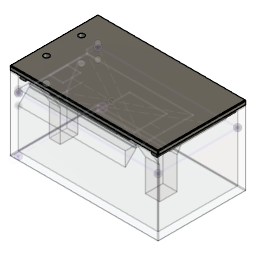
ESP32_case_v2 (Autodesk Fusion 360 design; units mm, degrees)
Autodesk Fusion 360 part; units mm, degrees
note: some values were not read from the file. Chosen so that the rebuilt part matches the saved one: a direction. Set by a fixed rule: which sketch regions a step uses.
sketch "Sketch1" plane through (0, 0, 0) normal (0, 0, 1) x (1, 0, 0) in component "Case bottom"
  line L0 (0, 0) -> (63.9, 0)
  line L1 (63.9, 0) -> (63.9, 36.4)
  line L2 (63.9, 36.4) -> (0, 36.4)
  line L3 (0, 36.4) -> (0, 0)
  line L4 (-2, -2) -> (65.9, -2)
  line L5 (65.9, -2) -> (65.9, 38.4)
  line L6 (65.9, 38.4) -> (-2, 38.4)
  line L7 (-2, 38.4) -> (-2, -2)
  dimension "d3" = 63.9
  dimension "d4" = 36.4
  dimension "d5" = 2
  constraint horizontal L0
  constraint vertical L1
  constraint horizontal L2
  constraint vertical L3
  constraint coincident L0.start L3.end
  measures "d3" distance of L0.start L0.end
  measures "d4" distance of L0.start L2.end
extrude "Extrude1" add sketch "Sketch1" along normal blind 2 contours L0 L1 L2 L3 | L4 L5 L6 L7 makes body 1 in component "Case bottom"
extrude "Extrude2" add sketch "Sketch1" along normal blind 34 bodies 1 in component "Case bottom"
sketch "Sketch2" plane through (0, 0, 0) normal (1, 0, 0) x (0, 1, 0) in component "Case bottom"
  line L0 (36.4, 2) -> (36.4, 34)
  line L1 (36.4, 34) -> (0, 34)
  line L2 (0, 34) -> (0, 2)
  line L3 (14.2, 0) -> (22.2, 0)
  line L4 (22.2, 0) -> (22.2, 14.6077)
  line L5 (22.2, 14.6077) -> (14.2, 14.6077)
  line L6 (14.2, 14.6077) -> (14.2, 0)
  line L7 (18.2, 14.6077) -> (18.2, 0) construction
  line L8 (-2, 0) -> (38.4, 0) construction
  line L9 (22.2, 14.6077) -> (28.2, 25)
  line L10 (22.2, 14.6077) -> (29.239, 14.6077) construction
  line L11 (14.2, 14.6077) -> (8.2, 25)
  line L12 (14.2, 14.6077) -> (29.239, 14.6077) construction
  line L13 (8.2, 25) -> (28.2, 25)
  line L14 (0, 2) -> (36.4, 2)
  line L15 (0, 20) -> (5, 25)
  line L16 (5, 25) -> (5, 26.5)
  line L17 (5, 26.5) -> (0, 26.5)
  line L18 (8.2, 25) -> (0, 25) construction
  line L19 (31.4, 26.5) -> (36.4, 26.5)
  line L20 (31.4, 25) -> (31.4, 26.5)
  line L21 (36.4, 20) -> (31.4, 25)
  dimension "d12" = 8
  dimension "d13" = 60
  dimension "d14" = 120
  dimension "d15" = 20
  dimension "d17" = 7.039
  dimension "d18" = 25
  dimension "d113" = 1.5
  dimension "d114" = 5
  dimension "d115" = 45
  constraint horizontal L3
  constraint vertical L4
  constraint horizontal L5
  constraint vertical L6
  constraint midpoint L5 L7.start
  constraint midpoint L3 L7.end
  constraint midpoint L7.end L8
  constraint horizontal L10
  constraint horizontal L12
  constraint horizontal L13
  constraint coincident L2 L15.start
  constraint parallel L2 L16
  constraint coincident L2 L17.end
  constraint perpendicular L2 L17
  constraint coincident L2 L18.end
  constraint perpendicular L2 L18
  constraint coincident L15.end L18
  constraint symmetric L7 L15.start L21.start
  constraint symmetric L7 L15.end L20.start
  constraint symmetric L7 L16.end L19.start
  constraint symmetric L7 L17.end L19.end
  measures "d12" distance of L4.end L5.end
  measures "d13" angle of L9 L10
  measures "d14" angle of L11 L12
  measures "d15" distance of L9.end L11.end
  measures "d17" distance of L4.end L10.end
  measures "d18" distance of L8 L11.end
  measures "d113" distance of L15.end L16.end
  measures "d114" distance of L16.end L17.end
  measures "d115" angle of L2 L15
extrude "Extrude3" add sketch "Sketch2" along normal blind 5 separate body contours L4 L5 L6 L14 | L3 L4 L6 L14 | L5 L9 L11 L13 makes body 2 in component "Case bottom"
fillet "Fillet1" radius 1 2 edges at (2.5, 28.2, 25) (2.5, 8.2, 25) on bodies 2 in component "Case bottom"
pattern_linear "R-Pattern1" count 2 spacing 43.9 along (1, 0, 0) of bodies 2 makes body 3 in component "Case bottom"
sketch "Sketch1 (2)" plane through (0, 0, 25) normal (0, 0, 1) x (-1, 0, 0) in component "board"
  line L0 (0, -9.9321) -> (-5, -9.9321)
  line L1 (-5, -9.9321) -> (-5, -26.4679)
  line L2 (-5, -26.4679) -> (0, -26.4679)
  line L3 (0, -26.4679) -> (0, -9.9321)
  line L4 (0, -36.4) -> (0, 0)
  line L5 (-63.9, -36.4) -> (0, -36.4)
  line L6 (-63.9, 0) -> (-63.9, -36.4)
  line L7 (0, 0) -> (-63.9, 0)
  line L8 (0, -36.4) -> (-63.9, 0) construction
  line L9 (-63.9, -36.4) -> (0, 0) construction
  line L10 (-48.7, -5.2) -> (-0.2, -5.2)
  line L11 (-0.2, -5.2) -> (-0.2, -31.2)
  line L12 (-0.2, -31.2) -> (-48.7, -31.2)
  line L13 (-48.7, -31.2) -> (-48.7, -5.2)
  line L14 (-48.7, -5.2) -> (-0.2, -31.2) construction
  line L15 (-0.2, -5.2) -> (-48.7, -31.2) construction
  line L16 (-25.2, -25.7) -> (-42.2, -25.7)
  line L17 (-42.2, -25.7) -> (-42.2, -10.7)
  line L18 (-42.2, -10.7) -> (-25.2, -10.7)
  line L19 (-25.2, -10.7) -> (-25.2, -25.7)
  line L20 (-42.2, -18.2) -> (-48.7, -18.2) construction
  line L21 (-0.2, -22.2) -> (-6.2, -22.2)
  line L22 (-6.2, -22.2) -> (-6.2, -14.2)
  line L23 (-6.2, -14.2) -> (-0.2, -14.2)
  line L24 (-0.2, -14.2) -> (-0.2, -22.2)
  line L25 (-6.2, -18.2) -> (-25.2, -18.2) construction
  circle A0 centre (-2.7, -26.2) radius 1.25
  circle A1 centre (-2.7, -10.2) radius 1.25
  point P0 (-24.45, -18.2)
  dimension "d32" = 48.5
  dimension "d33" = 26
  dimension "d85" = 17
  dimension "d86" = 15
  dimension "d87" = 6.5
  dimension "d89" = 6
  dimension "d90" = 8
  dimension "d124" = 2.5
  dimension "d125" = 2.5
  dimension "d126" = 5
  dimension "d127" = 5
  dimension "d128" = 2.5
  dimension "d129" = 2.5
  dimension "d141" = 5.2
  dimension "d142" = 0.2
  constraint coincident L4.start L5.end
  constraint coincident L6.start L7.end
  constraint coincident L5.start L6.end
  constraint coincident L4.end L7.start
  constraint horizontal L10
  constraint perpendicular L10 L11
  constraint parallel L10 L12
  constraint parallel L11 L13
  constraint coincident L14 P0
  constraint coincident L15 P0
  constraint horizontal L16
  constraint vertical L17
  constraint horizontal L18
  constraint vertical L19
  constraint midpoint L17 L20.start
  constraint midpoint L13 L20.end
  constraint horizontal L20
  constraint horizontal L21
  constraint vertical L22
  constraint horizontal L23
  constraint vertical L24
  constraint coincident L11 L21.start
  constraint midpoint L22 L25.start
  constraint midpoint L19 L25.end
  constraint horizontal L25
  measures "d32" distance of L11.end L12.end
  measures "d33" distance of L10.end L11.end
  measures "d85" distance of L16.start L16.end
  measures "d86" distance of L16.start L18.end
  measures "d87" distance of L13 L17
  measures "d89" distance of L21.start L21.end
  measures "d90" distance of L21.start L23.end
  measures "d124" distance of L11 A0.centre
  measures "d125" distance of L11 A1.centre
  measures "d126" distance of L12 A0.centre
  measures "d127" distance of L10 A1.centre
  measures "d128" diameter of A0
  measures "d129" diameter of A1
  measures "d141" distance of L5 L12
  measures "d142" distance of L4 L11
extrude "Extrude2'" add sketch "Sketch1 (2)" along normal blind 1.54 separate body contours L0 L1 L11 L23 A1 | L0 L1 L2 L10 L11 L12 L13 L21 L22 L23 A0 A1 | L0 A1 | L0 A1 | L1 L11 L21 L23 L24 | L1 L2 L11 L21 A0 | L1 L21 L22 L23 | L2 A0 | L2 A0 | L16 L17 L18 L19 makes body 4 in component "board"
sketch "Sketch2 (2)" plane through (0.2, 0, 0) normal (-1, 0, 0) x (0, -1, 0) in component "board"
  line L0 (-31.2, 25) -> (-5.2, 25)
  line L1 (-5.2, 25) -> (-5.2, 26.54)
  line L2 (-5.2, 26.54) -> (-31.2, 26.54)
  line L3 (-31.2, 26.54) -> (-31.2, 25)
  line L4 (-22.7, 26.54) -> (-13.7, 26.54)
  line L5 (-13.7, 26.54) -> (-13.7, 29.56)
  line L6 (-13.7, 29.56) -> (-22.7, 29.56)
  line L7 (-22.7, 29.56) -> (-22.7, 26.54)
  dimension "d36" = 9
  dimension "d37" = 3.02
  constraint horizontal L4
  constraint vertical L5
  constraint horizontal L6
  constraint vertical L7
  constraint coincident L2 L4.start
  constraint midpoint L2 L4
  measures "d36" distance of L4.start L4.end
  measures "d37" distance of L4.start L6.end
extrude "Extrude3'" add sketch "Sketch2 (2)" along normal blind 2.2 and the other way blind 6 contours L2 L4 L5 L6 L7 bodies 4 in component "board"
fillet "Fillet1'" radius 1 4 edges at (2.1, 13.7, 29.56) (-0.9, 13.7, 26.54) (2.1, 22.7, 29.56) (-0.9, 22.7, 26.54) on bodies 4 in component "board"
sketch "Sketch3" plane through (-2, 0, 0) normal (-1, 0, 0) x (0, -1, 0) in component "Case bottom"
  line L0 (-38.4, 0) -> (2, 0)
  line L1 (2, 0) -> (2, 34)
  line L2 (2, 34) -> (-38.4, 34)
  line L3 (-38.4, 34) -> (-38.4, 0)
  arc A0 (-22.7, 27.54) -> (-21.7, 26.54) centre (-21.7, 27.54) ccw
  line L4 (-21.7, 26.54) -> (-14.7, 26.54)
  arc A1 (-14.7, 26.54) -> (-13.7, 27.54) centre (-14.7, 27.54) ccw
  line L5 (-13.7, 27.54) -> (-13.7, 28.56)
  arc A2 (-13.7, 28.56) -> (-14.7, 29.56) centre (-14.7, 28.56) ccw
  line L6 (-14.7, 29.56) -> (-21.7, 29.56)
  arc A3 (-21.7, 29.56) -> (-22.7, 28.56) centre (-21.7, 28.56) ccw
  line L7 (-22.7, 28.56) -> (-22.7, 27.54)
  line L8 (-23.7, 28.56) -> (-23.7, 27.54)
  arc A4 (-23.7, 27.54) -> (-21.7, 25.54) centre (-21.7, 27.54) ccw
  line L9 (-21.7, 25.54) -> (-14.7, 25.54)
  arc A5 (-14.7, 25.54) -> (-12.7, 27.54) centre (-14.7, 27.54) ccw
  line L10 (-12.7, 27.54) -> (-12.7, 28.56)
  arc A6 (-12.7, 28.56) -> (-14.7, 30.56) centre (-14.7, 28.56) ccw
  line L11 (-14.7, 30.56) -> (-21.7, 30.56)
  arc A7 (-21.7, 30.56) -> (-23.7, 28.56) centre (-21.7, 28.56) ccw
  dimension "d44" = 1
extrude "Extrude4" cut sketch "Sketch3" against normal blind 2 contours A0 L4 A1 L5 A2 L6 A3 L7 | L8 A4 L9 A5 L10 A6 L11 A7 bodies 1 in component "Case bottom"
sketch "Sketch1 (3)" plane through (0, 0, 34) normal (0, 0, 1) x (-1, 0, 0) in component "Lid"
  line L0 (0, 0) -> (0, -36.4)
  line L1 (0, -36.4) -> (-63.9, -36.4)
  line L2 (-63.9, -36.4) -> (-63.9, 0)
  line L3 (-63.9, 0) -> (0, 0)
  line L4 (2, -38.4) -> (2, 2)
  line L5 (2, 2) -> (-65.9, 2)
  line L6 (-65.9, 2) -> (-65.9, -38.4)
  line L7 (-65.9, -38.4) -> (2, -38.4)
  line L8 (-13.95, -36.2) -> (-49.95, -36.2)
  line L9 (-49.95, -36.2) -> (-49.95, -33.2)
  line L10 (-49.95, -33.2) -> (-13.95, -33.2)
  line L11 (-13.95, -33.2) -> (-13.95, -36.2)
  line L12 (-63.9, -36.4) -> (0, -36.4)
  line L13 (-31.95, -36.2) -> (-31.95, -33.2) construction
  line L14 (0, -36.4) -> (0, 0) construction
  line L15 (-63.9, 0) -> (-63.9, -36.4) construction
  line L16 (-38.9, -22.2) -> (-30.9, -22.2)
  line L17 (-30.9, -22.2) -> (-30.9, -14.2)
  line L18 (-30.9, -14.2) -> (-38.9, -14.2)
  line L19 (-38.9, -14.2) -> (-38.9, -22.2)
  line L20 (-38.9, -18.2) -> (-63.9, -18.2) construction
  line L21 (-6, -22.2) -> (-3, -22.2)
  line L22 (-3, -22.2) -> (-3, -14.2)
  line L23 (-3, -14.2) -> (-6, -14.2)
  line L24 (-6, -14.2) -> (-6, -22.2)
  line L25 (-6, -18.2) -> (-30.9, -18.2) construction
  circle A0 centre (-2.7, -10.2) radius 1.25
  circle A1 centre (-2.7, -26.2) radius 1.25
  point P0 (-2.7, -10.2)
  point P1 (-2.7, -26.2)
  dimension "d51" = 0.2
  dimension "d52" = 36
  dimension "d53" = 3
  dimension "d54" = 31.95
  dimension "d55" = 13.95
  dimension "d59" = 13.95
  dimension "d95" = 8
  dimension "d96" = 8
  dimension "d97" = 25
  dimension "d98" = 3
  dimension "d99" = 8
  dimension "d100" = 3
  constraint horizontal L8
  constraint vertical L9
  constraint horizontal L10
  constraint vertical L11
  constraint midpoint L8 L13.start
  constraint midpoint L10 L13.end
  constraint horizontal L16
  constraint vertical L17
  constraint horizontal L18
  constraint vertical L19
  constraint midpoint L19 L20.start
  constraint midpoint L2 L20.end
  constraint horizontal L20
  constraint horizontal L21
  constraint vertical L22
  constraint horizontal L23
  constraint vertical L24
  constraint midpoint L24 L25.start
  constraint midpoint L17 L25.end
  constraint horizontal L25
  measures "d51" distance of L8 L12
  measures "d52" distance of L9.end L10.end
  measures "d53" distance of L8.start L10.end
  measures "d54" distance of L13 L14
  measures "d55" distance of L11 L14
  measures "d59" distance of L9 L15
  measures "d95" distance of L16.start L16.end
  measures "d96" distance of L16.start L18.end
  measures "d97" distance of L2 L19
  measures "d98" distance of L21.start L21.end
  measures "d99" distance of L21.start L23.end
  measures "d100" distance of L14 L22
extrude "Extrude1'" add sketch "Sketch1 (3)" along normal blind 2 separate body contours L0 L1 L2 L3 L12 | L4 L5 L6 L7 | L8 L9 L10 L11 | L16 L17 L18 L19 | L21 L22 L23 L24 | A0 | A1 makes body 5 in component "Lid"
extrude "Extrude2''" add sketch "Sketch1 (3)" against normal blind 3 separate body contours L8 L9 L10 L11 makes body 6 in component "Lid"
sketch "Sketch2 (3)" plane through (13.95, 0, 0) normal (-1, 0, 0) x (0, -1, 0) in component "Lid"
  line L0 (-33.2, 34) -> (-36.2, 34)
  line L1 (-36.2, 34) -> (-36.2, 31)
  line L2 (-36.2, 31) -> (-33.2, 31)
  line L3 (-33.2, 31) -> (-33.2, 34)
  line L4 (-36.2, 31) -> (-35.4929, 31.7071)
  line L5 (-35.4929, 31.7071) -> (-35.4929, 32.7929)
  line L6 (-36.2, 34) -> (-36.2, 33.5)
  line L7 (-35.4929, 32.7929) -> (-36.2, 33.5)
  dimension "d65" = 1
  dimension "d67" = 135
  dimension "d68" = 0.5
  dimension "d69" = 135
  constraint coincident L1.end L2.start
  constraint perpendicular L2 L5
  constraint coincident L0.end L1.start
  constraint perpendicular L0 L6
  measures "d65" distance of L1.end L4.end
  measures "d67" angle of L4 L5
  measures "d68" distance of L0.end L6.end
  measures "d69" angle of L5 L7
extrude "Extrude3''" cut sketch "Sketch2 (3)" against normal up to surface (36 mm away) contours L1 L4 L5 L7 bodies 6 in component "Lid"
fillet "Fillet1''" radius 0.2 2 edges at (31.95, 36.2, 31) (31.95, 33.2, 31) on bodies 6 in component "Lid"
pattern_path "PathPattern1" count 4 spacing 50.15 from (31.95, 36.4, 34) turning path "Sketch1 (3)" along L3 L0 L1 L2 of bodies 6 makes body 7 at (62.7, 24.2, 34) makes body 8 at (37.95, 1.2, 34) makes body 9 at (1.2, 12.2, 34) in component "Lid"
sketch "Sketch4" plane through (13.95, 0, 0) normal (-1, 0, 0) x (0, -1, 0) in component "Case bottom"
  arc A0 (-33.4, 31) -> (-33.2, 31.2) centre (-33.4, 31.2) ccw
  line L0 (-33.2, 31.2) -> (-33.2, 34)
  line L1 (-33.2, 34) -> (-36.2, 34)
  line L2 (-36.2, 34) -> (-36.2, 33.5)
  line L3 (-36.2, 33.5) -> (-35.4929, 32.7929)
  line L4 (-35.4929, 32.7929) -> (-35.4929, 31.7071)
  line L5 (-35.4929, 31.7071) -> (-35.8586, 31.3414)
  arc A1 (-35.8586, 31.3414) -> (-35.7172, 31) centre (-35.7172, 31.2) ccw
  line L6 (-35.7172, 31) -> (-33.4, 31)
  line L7 (-36.4, 34) -> (-36.4, 33.4172)
  line L8 (-36.4, 33.4172) -> (-35.6929, 32.7101)
  line L9 (-35.6929, 32.7101) -> (-35.6929, 31.7899)
  line L10 (-35.6929, 31.7899) -> (-36.4, 31.0828)
  line L11 (-36.4, 2) -> (-36.4, 34)
  dimension "d75" = 0.2
  dimension "d77" = 0.5828
  constraint coincident L10.end L11
  measures "d77" distance of L7.start L7.end
extrude "Extrude5" add sketch "Sketch4" against normal blind 26 from surface at -5 separate body contours L8 L9 L10 L11 makes body 10 in component "Case bottom"
fillet "Fillet2" radius 0.3 2 edges at (31.95, 35.6929, 32.7101) (31.95, 35.6929, 31.7899) on bodies 10 in component "Case bottom"
pattern_path "PathPattern1'" count 4 spacing 50.15 from (31.95, 36.4, 34) turning along 4 edges at (31.95, 36.4, 34) (63.9, 18.2, 34) (31.95, 0, 34) (0, 18.2, 34) of bodies 10 on bodies 1 makes body 11 at (63.9, 22.5333, 31.8609) makes body 12 at (36.2833, 0, 31.8609) makes body 13 at (0, 13.8667, 31.8609) in component "Case bottom"
extrude "Extrude5'" add sketch "Sketch1 (2)" along normal blind 4.75 separate body contours L16 L17 L18 L19 makes body 14 in component "board"
extrude "Extrude6" add sketch "Sketch1 (2)" along normal blind 2.54 contours L0 A1 | L0 A1 | L2 A0 | L2 A0 bodies 4 in component "board"
extrude "Extrude4'" add sketch "Sketch1 (3)" against normal blind 4.05 separate body contours L16 L17 L18 L19 | L21 L22 L23 L24 makes body 15 at (36.2333, 19.5333, 34) makes body 16 at (6, 16.8667, 32.65) in component "Lid"
fillet "Fillet2'" radius 0.3 12 edges at (-2, -2, 35) (-2, 18.2, 36) (-2, 18.2, 34) (31.95, -2, 36) (31.95, -2, 34) (65.9, -2, 35) (65.9, 18.2, 36) (65.9, 18.2, 34) (65.9, 38.4, 35) (31.95, 38.4, 36) (31.95, 38.4, 34) (-2, 38.4, 35) on bodies 5 in component "Lid"
fillet "Fillet3" radius 0.3 8 edges at (30.9, 18.2, 29.95) (34.9, 14.2, 29.95) (34.9, 22.2, 29.95) (38.9, 18.2, 29.95) (4.5, 14.2, 29.95) (6, 18.2, 29.95) (4.5, 22.2, 29.95) (3, 18.2, 29.95) on bodies 15 16 in component "Lid"
extrude "Extrude5''" cut sketch "Sketch1 (3)" along normal up to surface (2 mm away) and the other way up to surface (3 mm away) contours A0 | A1 bodies 5 9 in component "Lid"
fillet "Fillet3'" radius 0.3 16 edges at (65.9, 38.4, 17) (65.9, -2, 17) (-2, -2, 17) (-2, 38.4, 17) (31.95, -2, 0) (-2, 18.2, 0) (31.95, 38.4, 0) (65.9, 18.2, 0) (31.95, -2, 34) (-2, 18.2, 34) (31.95, 38.4, 34) (0, 18.2, 34) (31.95, 36.4, 34) (31.95, 0, 34) (65.9, 18.2, 34) (63.9, 18.2, 34) on bodies 1 in component "Case bottom"
extrude "Extrude6'" add sketch "Sketch2" along normal blind 48.9 contours L0 L19 L20 L21 | L2 L15 L16 L17 bodies 1 in component "Case bottom"
move_face "OffsetFaces1" offset 1.5 1 faces at (48.9, 16.8667, 21.5359) on bodies 3 in component "Case bottom"
sketch "Sketch5" plane through (0, 0, 25) normal (0, 0, 1) x (-1, 0, 0) in component "Case bottom"
  line L0 (-43.9, -9.9321) -> (-50.4, -9.9321)
  line L1 (-50.4, -9.9321) -> (-50.4, -26.4679)
  line L2 (-50.4, -26.4679) -> (-43.9, -26.4679)
  line L3 (-43.9, -26.4679) -> (-43.9, -9.9321)
  line L4 (-50.4, -26.4679) -> (-48.9, -26.4679)
  line L5 (-48.9, -26.4679) -> (-48.9, -9.9321)
  line L6 (-48.9, -9.9321) -> (-50.4, -9.9321)
  line L7 (-50.4, -9.9321) -> (-50.4, -26.4679)
  dimension "d119" = 1.5
  constraint horizontal L4
  constraint vertical L5
  constraint horizontal L6
  constraint vertical L7
  constraint coincident L0 L5.end
  constraint coincident L1.end L2.start
  measures "d119" distance of L5.end L0.end
extrude "Extrude7" add sketch "Sketch5" along normal blind 1.5 contours L0 L1 L2 L4 L5 L6 L7 bodies 3 in component "Case bottom"
fillet "Fillet5" radius 0.3 8 edges at (24.45, 31.4, 26.5) (24.45, 5, 26.5) (24.45, 31.4, 25) (24.45, 5, 25) (48.9, 18.2, 26.5) (49.65, 26.4679, 26.5) (49.65, 9.9321, 26.5) (50.4, 18.2, 26.5) on bodies 1 3 in component "Case bottom"
component "Case bottom" placed x (1, 0, 0) y (0, 1, 0) z (0, 0, 1) at (0, 0, 0)
component "board" placed x (1, 0, 0) y (0, 1, 0) z (0, 0, 1) at (0, 0, 0)
component "Lid" placed x (1, 0, 0) y (0, 1, 0) z (0, 0, 1) at (0, 0, 0)
equation "d3 = length + tolerance * 2"
equation "d4 = width + tolerance * 2"
equation "wall = 2 mm"
equation "d7 = wall"
equation "d9 = wall + height"
equation "height = 32 mm"
equation "d14 = 90 deg + 30 deg"
equation "d18 = wall + board_height"
equation "d25 = -( length + tolerance * 2 ) + 5 mm + length_space"
equation "length = board_length + length_space"
equation "width = board_width + width_space"
equation "tolerance = 0.2 mm"
equation "d32 = length - 15 mm"
equation "d33 = width - 10 mm"
equation "d34 = board_thicknes"
equation "d45 = -wall"
equation "d47 = -wall"
equation "d49 = wall"
equation "d51 = tolerance"
equation "d52 = width"
equation "d54 = ( length + tolerance * 2 ) / 2"
equation "d63 = path"
equation "path = ( length + tolerance * 2 ) / 2 + length + tolerance * 2 + width + tolerance * 2 + ( width + tolerance * 2 ) / 2"
equation "d75 = tolerance"
equation "d78 = -width + 5 mm + 5 mm"
equation "d83 = path"
equation "board_height = 23 mm"
equation "board_thicknes = 1.54 mm"
equation "d93 = board_chip_thicknes"
equation "d97 = 10 mm + 15 mm"
equation "d101 = -( height - board_height - board_chip_thicknes - tolerance )"
equation "board_chip_thicknes = 4.75 mm"
equation "d116 = length + tolerance * 2 - 15 mm"
equation "d132 = board_thicknes + 1 mm"
equation "length_space = 15 mm"
equation "width_space = 10 mm"
equation "board_length = 48.5 mm"
equation "board_width = 26 mm"
